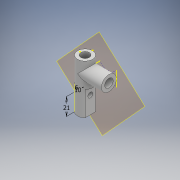
# Autodesk Inventor part: basechassis
Saved by Autodesk Inventor 2018 (Build 220112000, 112)
## iProperties
Created: 2018-11-21
Part Number: basechassis
Material: Generic
Document SubType Name: Modeling
Designer: Prakash
Density: 1 g/cm^3
Appearance: Default
Author: Prakash
Autodesk Inventor part; units mm, degrees
ref_plane "YZ Plane" through (0, 0, 0) normal (1, 0, 0) x (0, 1, 0)
ref_plane "XZ Plane" through (0, 0, 0) normal (0, 1, 0) x (-1, 0, 0)
ref_plane "XY Plane" through (0, 0, 0) normal (0, 0, 1) x (1, 0, 0)
sketch "Sketch1" plane through (0, 0, 0) normal (0, 0, 1) x (1, 0, 0)
  circle A0 centre (0, 0) radius 5.125
  circle A1 centre (0, 0) radius 9.125
  dimension "d0" = 10.25
  dimension "d1" = 18.25
  constraints: 2 centre point, 2 coincident
  measures "d0" diameter of A0
  measures "d1" diameter of A1
extrude "Extrusion1" add sketch "Sketch1" against normal blind 30
sketch "Sketch2" plane through (0, 0, -30) normal (0, 0, -1) x (-1, 0, 0)
  circle A0 centre (0, 0) radius 5.125 projected
  circle A1 centre (0, 0) radius 9.125 projected
  circle A2 centre (0, 0) radius 9.125 projected
  arc A3 (6.4043, 6.5) -> (-6.4043, 6.5) centre (0, 0) ccw
  arc A4 (-6.4043, -6.5) -> (6.4043, -6.5) centre (0, 0) ccw
  line L0 (-6.4043, 6.5) -> (-6.4043, -6.5)
  line L1 (6.4043, 6.5) -> (6.4043, -6.5)
  line L2 (0, 9.125) -> (0, -9.125) construction
  dimension "d4" = 13
  constraints: 12 point on circle, 6 end point, 3 vertical, 2 centre point, 1 midpoint
  measures "d4" distance of L1.start L1.end
extrude "Extrusion2" add sketch "Sketch2" along normal blind 30 contours A0 | L1 A1 L0
ref_plane "Work Plane1" through (9.125, 0, 0) normal (1, 0, 0) x (0, 1, 0)
sketch "Sketch3" plane through (9.125, 0, 0) normal (1, 0, 0) x (0, 1, 0)
  line L0 (9.125, 0) -> (9.125, -60) projected
  line L1 (-9.125, 0) -> (-9.125, -60) projected
  circle A0 centre (0, -15.1245) radius 9.125
  line L2 (9.125, -15.1245) -> (0, -15.1245) construction
  line L3 (0, -15.1245) -> (-9.125, -15.1245) construction
  line L4 (-9.125, 0) -> (9.125, 0) construction
  circle A1 centre (0, -15.1245) radius 5.125
  point P0 (0, 0)
  dimension "d7" = 15.1245
  dimension "d8" = 10.25
  constraints: 4 end point, 3 point on line, 1 centre point, 1 coincident, 1 collinear, 1 horizontal, 1 horizontal alignment, 2 other
  measures "d7" distance from line of L4 L2.end
  measures "d8" diameter of A1
extrude "Extrusion3" add sketch "Sketch3" against normal up to surface contours A0 | A1 round surface about axis through (0, 0, 0) along (0, 0, -1) radius 9.125 far side no
extrude "Extrusion4" add sketch "Sketch3" along normal blind 20
sketch "Sketch4" plane through (-6.4043, -6.5, -30) normal (-1, 0, 0) x (0, 0, 1)
  circle A0 centre (-9, 6.5) radius 5
  line L0 (0, 13) -> (0, 0) projected
  line L1 (0, 13) -> (-30, 13) projected
  line L2 (-30, 0) -> (-30, 13) projected
  line L3 (0, 0) -> (-30, 0) projected
  line L4 (-9, 13) -> (-9, 6.5) construction
  line L5 (-9, 6.5) -> (-9, 0) construction
  circle A1 centre (-9, 6.5) radius 3
  point P0 (30, 6.5)
  dimension "d13" = 10
  dimension "d14" = 21
  dimension "d15" = 6
  constraints: 4 end point, 3 point on line, 2 centre point, 1 coincident, 1 collinear, 1 vertical
  measures "d13" diameter of A0
  measures "d14" distance from line of L2 L4.end
  measures "d15" diameter of A1
extrude "Extrusion5" cut sketch "Sketch4" against normal blind 4 contours A0 | A1
extrude "Extrusion6" cut sketch "Sketch4" against normal up to surface (12.8087 mm away) contours A1
ref_plane "Work Plane3" through (9.125, 9.125, 0) normal (0, 1, 0) x (-1, 0, 0)
sketch "Sketch6" plane through (9.125, 9.125, 0) normal (0, 1, 0) x (-1, 0, 0)
  line L0 (0, -24.2495) -> (9.125, -15.1245) projected
  line L1 (9.125, -15.1245) -> (0, -5.9995) projected
  line L2 (-20, -5.9995) -> (-20, -24.2495) projected
  line L3 (0, -5.9995) -> (-20, -24.2495) construction
  line L4 (0, -24.2495) -> (-20, -5.9995) construction
  point P0 (9.125, 0)
  point P1 (-10, -15.1245)
  constraints: 4 end point, 1 coincident, 1 midpoint
ref_plane "Work Plane4" through (9.125, 9.125, -5.9995) normal (0, -1, 0) x (0.7386854, 0, -0.6740504)
sketch "Sketch7" plane through (9.125, 9.125, -5.9995) normal (0, -1, 0) x (0.7386854, 0, -0.6740504)
  line L0 (12.3014, -13.481) -> (14.7737, 13.481) construction
  line L1 (0, 0) -> (27.0751, 0) construction
  line L2 (27.0751, 0) -> (14.7737, 13.481) projected
  line L3 (-0.5898, -12.8912) -> (-0.5898, -12.8912) projected
  line L4 (-0.5898, -12.8912) -> (-0.5898, -12.8912) projected
  circle A0 centre (13.5376, 0) radius 2.5275
  point P0 (-10.7845, -1.719)
  dimension "d20" = 5.055
  constraints: 1 centre point, 1 coincident
  measures "d20" diameter of A0
extrude "Extrusion7" cut sketch "Sketch7" along normal blind 3.81
sketch "Sketch9" plane through (9.125, 9.125, -5.9995) normal (0, -1, 0) x (0.7386854, 0, -0.6740504)
  line L0 (0, 0) -> (27.0751, 0) construction
  line L1 (12.3014, -13.481) -> (14.7737, 13.481) construction
  circle A0 centre (13.5376, 0) radius 2.6545
  point P0 (-10.7845, -1.719)
  dimension "d24" = 5.309
  constraints: 1 centre point, 1 coincident
  measures "d24" diameter of A0
loft "Loft1" cut profiles "Sketch9" section 1 edges at (17.258, 5.315, -13.4208)
sketch "Sketch10" plane through (19.125, 5.315, -15.1245) normal (0, 1, 0) x (1, 0, 0)
  line L0 (-10, 9.125) -> (10, -9.125) construction
  line L1 (-10, -9.125) -> (10, 9.125) construction
  circle A0 centre (0, 0) radius 1.8
  point P0 (-19.125, -15.1245)
  dimension "d29" = 3.6
  constraints: 1 centre point, 1 coincident
  measures "d29" diameter of A0
extrude "Extrusion8" cut sketch "Sketch10" against normal up to surface round surface about axis through (9.125, 0, -15.1245) along (1, 0, 0) radius 5.125 far side no
body "Solid1"
